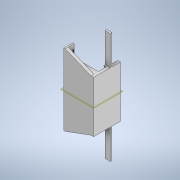
# Autodesk Inventor part: gira
Saved by Autodesk Inventor 2020 (Build 240168000, 168)
## iProperties
Created: 2022-10-31
Part Number: gira
Material: Generic
Document SubType Name: Modeling
Designer: super
Density: 1 g/cm^3
Appearance: Default
Author: super
Autodesk Inventor part; units mm, degrees
ref_plane "YZ Plane" through (0, 0, 0) normal (1, 0, 0) x (0, 1, 0)
ref_plane "XZ Plane" through (0, 0, 0) normal (0, 1, 0) x (-1, 0, 0)
ref_plane "XY Plane" through (0, 0, 0) normal (0, 0, 1) x (1, 0, 0)
ref_plane "Work Plane1" through (-84.567877, -177.761364, 10.407851) normal (0.999999, 0.0014131, 0) x (0.0014131, -0.999999, 0)
sketch "Sketch1" plane through (-84.567877, -177.761364, 10.407851) normal (0.999999, 0.0014131, 0) x (0.0014131, -0.999999, 0)
  line L0 (9.629544, -13.988982) -> (-230.370456, -13.988982)
  line L1 (-230.370456, -13.988982) -> (-230.370456, 6.011018)
  line L2 (-230.370456, 6.011018) -> (9.629544, 6.011018)
  line L3 (9.629544, 6.011018) -> (9.629544, -13.988982)
  point P0 (-177.641685, 10.407851)
  dimension "d40" = 240
  dimension "d41" = 20
  constraints: 8 end point, 2 parallel, 1 horizontal, 1 perpendicular
  measures "d40" distance of L0.start L0.end
  measures "d41" distance of L2.end L0.start
extrude "Extrusion1" add sketch "Sketch1" along normal blind 5
ref_plane "Work Plane2" through (-84.723841, -67.391019, 24.396834) normal (-0.0014131, 0.999999, 0) x (0.999999, 0.0014131, 0)
sketch "Sketch3" plane through (-84.55427, -187.390899, 24.396834) normal (0, 0, 1) x (0.999999, 0.0014131, 0)
  line L0 (0, 0) -> (5, 0)
  line L1 (5, 0) -> (91.254418, 31.830556)
  line L2 (91.254418, 31.830556) -> (100.362287, 31.830556)
  line L3 (100.362287, 31.830556) -> (100.362287, 204.349994)
  line L4 (100.362287, 204.349994) -> (91.254418, 204.349994)
  line L5 (5, 0) -> (5, 240)
  line L6 (91.254418, 204.349994) -> (5, 240)
  line L7 (0, 0) -> (0, 240)
  line L8 (5, 240) -> (0, 240)
  line L9 (0, 240) -> (0, 0)
  point P0 (84.818986, 187.271229)
  dimension "d42" = 172.51944
  dimension "d43" = 35.65001
  constraints: 16 end point, 3 perpendicular, 2 parallel, 1 horizontal
  measures "d42" distance of L2.end L3.end
  measures "d43" vertical distance of L4.end L5.end
extrude "Extrusion2" add sketch "Sketch3" along normal blind 10
sketch "Sketch4" plane through (-84.55427, -187.390899, 24.396834) normal (0, 0, -1) x (-0.999999, -0.0014131, 0)
  line L0 (-100.362287, 204.349994) -> (-91.254418, 204.349994)
  line L1 (-91.254418, 31.830556) -> (-100.362287, 31.830556)
  line L2 (-100.362287, 204.349994) -> (-91.254418, 204.349994)
  line L3 (-91.254418, 204.349994) -> (-91.254418, 31.830556)
  line L4 (-91.254418, 31.830556) -> (-100.362287, 31.830556)
  line L5 (-100.362287, 31.830556) -> (-100.362287, 204.349994)
  point P0 (-84.818986, 187.271229)
  point P1 (-100.362287, 31.830556)
  point P2 (-91.254418, 204.349994)
  constraints: 8 end point, 2 parallel, 1 horizontal, 1 perpendicular
extrude "Extrusion3" add sketch "Sketch4" along normal blind 80
sketch "Sketch6" plane through (15.762937, -155.418554, -55.603166) normal (0.0014131, -0.999999, 0) x (0.999999, 0.0014131, 0)
  line L0 (0, 0) -> (0, 90)
  line L1 (0, 28.554794) -> (0, 34.18669)
  line L2 (0, 34.18669) -> (-17.310634, 34.18669)
  line L3 (-17.310634, 34.18669) -> (-17.310634, 28.554794)
  line L4 (-17.310634, 28.554794) -> (0, 28.554794)
  point P0 (-15.5433, 55.603166)
  constraints: 8 end point, 2 parallel, 2 point on line, 1 perpendicular
extrude "Extrusion5" add sketch "Sketch6" along normal blind 100
sketch "Sketch7" plane through (6.655078, -155.431424, -27.048372) normal (0, 0, -1) x (-0.999999, -0.0014131, 0)
  line L0 (8.202765, 0) -> (0, 14.724355)
  line L1 (0, 172.519438) -> (0, 0)
  line L2 (8.202765, 0) -> (0, 0)
  line L3 (0, 0) -> (8.202765, 0)
  constraints: 4 end point, 1 collinear, 1 point on line
extrude "Extrusion6" add sketch "Sketch7" against normal blind 10
ref_plane "Work Plane3" through (15.641044, -69.158921, 34.396834) normal (-0.0014131, 0.999999, 0) x (0.999999, 0.0014131, 0)
mirror "Mirror1" about plane through (15.641044, -69.158921, 34.396834) normal (-0.0014131, 0.999999, 0) of "Extrusion5", "Extrusion6"
ref_plane "Work Plane4" through (-84.723841, -67.391019, 4.396834) normal (0.0014131, -0.999999, 0) x (0.999999, 0.0014131, 0)
sketch "Sketch10" plane through (-79.567882, -177.754299, 10.407851) normal (0.999999, 0.0014131, 0) x (0, 0, -1)
  point P0 (10.407851, 177.641685)
sketch "Sketch11" plane through (6.655078, -155.431424, -55.603166) normal (-0.999999, -0.0014131, 0) x (0, 0, 1)
  line L0 (80, 172.519438) -> (80, 0)
  line L1 (80, 172.519438) -> (64.947502, 172.519438)
  line L2 (64.947502, 172.519438) -> (64.947502, 165.746345)
  line L3 (64.947502, 165.746345) -> (80, 165.746345)
  line L4 (80, 165.746345) -> (80, 172.519438)
  point P0 (55.603166, 155.440673)
  point P1 (80, 165.746345)
  constraints: 8 end point, 2 parallel, 1 horizontal, 1 perpendicular
extrude "Extrusion7" add sketch "Sketch11" along normal blind 86.254
pattern_linear "Rectangular Pattern1" count 6 spacing 33 along (0.0014131, -0.999999, 0) of "Extrusion7"
sketch "Sketch14" plane through (-84.567877, -177.761364, 10.407851) normal (-0.999999, -0.0014131, 0) x (0, 0, 1)
  line L0 (23.988982, 230.370456) -> (23.988982, -9.629544)
  line L1 (-6.011018, -9.629544) -> (23.988982, -9.629544)
  point P0 (-10.407851, 177.641685)
  point P1 (-1.011018, 10.370456)
  dimension "d38" = 25
  dimension "d39" = 20
  measures "d38" distance from line of L0 point (-1.011, 10.37)
  measures "d39" distance from line of L1 point (-1.011, 10.37)
hole "Hole2" at (-84.582532, -167.390919, 9.396834) direction (0.999999, 0.0014131, 0) diameter 10 depth 8 tip angle 118
mirror "Mirror2" about plane through (-84.723841, -67.391019, 4.396834) normal (0.0014131, -0.999999, 0) of "Hole2"
body "Solid1"
